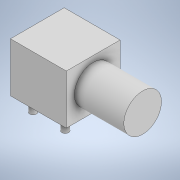
# Autodesk Inventor part: EPL.0s.302.HLN
Saved by Autodesk Inventor 2022 (Build 260153000, 153)
## iProperties
Created: 2022-03-03
Part Number: EPL.0s.302.HLN
Material: Generic
Document SubType Name: Modeling
Designer: elmar
Density: 1 g/cm^3
Appearance: Default
Author: elmar
Autodesk Inventor part; units mm, degrees
ref_plane "YZ Plane" through (0, 0, 0) normal (1, 0, 0) x (0, 1, 0)
ref_plane "XZ Plane" through (0, 0, 0) normal (0, 1, 0) x (-1, 0, 0)
ref_plane "XY Plane" through (0, 0, 0) normal (0, 0, 1) x (1, 0, 0)
sketch "Sketch1" plane through (0, 0, 0) normal (0, 0, 1) x (1, 0, 0)
  line L0 (6.604, -5.842) -> (-6.604, -5.842)
  line L1 (-6.604, -5.842) -> (-6.604, 5.842)
  line L2 (-6.604, 5.842) -> (6.604, 5.842)
  line L3 (6.604, 5.842) -> (6.604, -5.842)
  line L4 (6.604, -5.842) -> (-6.604, 5.842) construction
  line L5 (-6.604, -5.842) -> (6.604, 5.842) construction
  point P0 (0, 0)
  dimension "d0" = 13.208
  dimension "d1" = 11.684
  constraints: 12 end point, 2 midpoint, 2 parallel, 1 horizontal, 1 perpendicular
  measures "d0" distance of L1.end L2.end
  measures "d1" distance of L0.end L1.end
extrude "Extrusion1" add sketch "Sketch1" along normal blind 12.7
sketch "Sketch2" plane through (6.604, -5.842, 0) normal (1, 0, 0) x (0, 0, -1)
  circle A0 centre (-6.35, 5.842) radius 4.445
  line L0 (0, 0) -> (-12.7, 0) projected
  line L1 (0, 0) -> (0, 11.684) projected
  point P0 (0, 5.842)
  point P1 (-6.35, 0)
  point P2 (0, 5.842)
  dimension "d4" = 8.89
  constraints: 2 midpoint, 1 centre point, 1 horizontal alignment, 1 vertical alignment
  measures "d4" diameter of A0
extrude "Extrusion2" add sketch "Sketch2" along normal blind 11.684
sketch "Sketch3" plane through (-6.604, -5.842, 0) normal (0, -1, 0) x (1, 0, 0)
  line L0 (10.414, 2.54) -> (2.794, 2.54)
  line L1 (2.794, 2.54) -> (2.794, 10.16)
  line L2 (2.794, 10.16) -> (10.414, 10.16)
  line L3 (10.414, 10.16) -> (10.414, 2.54)
  line L4 (0, 0) -> (13.208, 0) projected
  line L5 (0, 0) -> (0, 12.7) projected
  circle A0 centre (10.414, 10.16) radius 0.8
  line L6 (7.874, 7.62) -> (7.874, 5.08)
  line L7 (7.874, 5.08) -> (5.334, 5.08)
  line L8 (5.334, 5.08) -> (5.334, 7.62)
  line L9 (5.334, 7.62) -> (7.874, 7.62)
  circle A1 centre (10.414, 2.54) radius 0.8
  circle A2 centre (5.334, 7.62) radius 0.8
  circle A3 centre (5.334, 5.08) radius 0.8
  circle A4 centre (2.794, 2.54) radius 0.8
  circle A5 centre (2.794, 10.16) radius 0.8
  point P0 (6.604, 0)
  point P1 (6.604, 6.35)
  point P2 (6.604, 0)
  point P3 (0, 6.35)
  point P4 (0, 6.35)
  point P5 (6.604, 6.35)
  point P6 (0, 6.35)
  point P7 (6.604, 0)
  point P8 (6.604, 0)
  dimension "d8" = 7.62
  dimension "d9" = 1.6
  dimension "d10" = 2.54
  constraints: 16 end point, 7 coincident, 6 centre point, 6 midpoint, 5 equal radius, 3 vertical alignment, 2 horizontal, 2 horizontal alignment, 18 other
  measures "d8" distance of L1.end L2.end
  measures "d9" diameter of A0
  measures "d10" distance of L8.end L6.start
extrude "Extrusion3" add sketch "Sketch3" along normal blind 3.2 contours A4 L1 L0 | L0 L1 A4 | A1 L3 L0 | L0 L3 A1 | A5 L2 L1 | L1 L2 A5 | A0 L2 L3 | L3 L2 A0 | A2 L8 L9 | L9 L8 A2 | A3 L8 L7 | L7 L8 A3
body "Solid1"
